Autodesk Fusion 360 part; units mm, degrees
(part 4 of 6)
  spline S19 degree 5 poles (-5.187272, -5.31052) (-5.191544, -5.314884) (-5.200224, -5.323457) (-5.213657, -5.335855) (-5.232349, -5.351511) (-5.256791, -5.369886) (-5.282015, -5.387403) (-5.307733, -5.404393) (-5.333731, -5.421097) (-5.359927, -5.437601) (-5.386324, -5.453892) (-5.412978, -5.469894) (-5.43996, -5.485516) (-5.467316, -5.500697) (-5.495045, -5.515434) (-5.523115, -5.52976) (-5.551479, -5.543728) (-5.580091, -5.55739) (-5.608915, -5.570786) (-5.637941, -5.583924) (-5.66717, -5.5968) (-5.69661, -5.609401) (-5.726271, -5.62171) (-5.756158, -5.633722) (-5.786265, -5.645438) (-5.816583, -5.656867) (-5.847101, -5.66802) (-5.877807, -5.678908) (-5.908693, -5.68954) (-5.939754, -5.699917) (-5.970988, -5.710041) (-6.002394, -5.71991) (-6.033972, -5.729522) (-6.065719, -5.738877) (-6.097633, -5.747977) (-6.129708, -5.756824) (-6.161942, -5.765422) (-6.194329, -5.773774) (-6.226867, -5.781881) (-6.259551, -5.789746) (-6.29238, -5.797368) (-6.325351, -5.804749) (-6.358463, -5.811889) (-6.391713, -5.818788) (-6.425099, -5.825448) (-6.458619, -5.831869) (-6.492269, -5.838053) (-6.526047, -5.844) (-6.55995, -5.849713) (-6.593977, -5.855191) (-6.628126, -5.860435) (-6.662394, -5.865445) (-6.69678, -5.870223) (-6.731281, -5.874768) (-6.765896, -5.879082) (-6.800622, -5.883164) (-6.835457, -5.887016) (-6.8704, -5.890638) (-6.905448, -5.89403) (-6.940601, -5.897193) (-6.975855, -5.900127) (-7.01121, -5.902834) (-7.046664, -5.905312) (-7.082214, -5.907563) (-7.117859, -5.909587) (-7.153598, -5.911384) (-7.189427, -5.912955) (-7.225345, -5.914299) (-7.26135, -5.915418) (-7.297442, -5.916311) (-7.33362, -5.916979) (-7.36263, -5.917334) (-7.384427, -5.917499) (-7.398975, -5.917564) (-7.406253, -5.917586) knots 0 0 0 0 0 0 0.01428571 0.02857143 0.04285714 0.05714286 0.07142857 0.08571429 0.1 0.11428571 0.12857143 0.14285714 0.15714286 0.17142857 0.18571429 0.2 0.21428571 0.22857143 0.24285714 0.25714286 0.27142857 0.28571429 0.3 0.31428571 0.32857143 0.34285714 0.35714286 0.37142857 0.38571429 0.4 0.41428571 0.42857143 0.44285714 0.45714286 0.47142857 0.48571429 0.5 0.51428571 0.52857143 0.54285714 0.55714286 0.57142857 0.58571429 0.6 0.61428571 0.62857143 0.64285714 0.65714286 0.67142857 0.68571429 0.7 0.71428571 0.72857143 0.74285714 0.75714286 0.77142857 0.78571429 0.8 0.81428571 0.82857143 0.84285714 0.85714286 0.87142857 0.88571429 0.9 0.91428571 0.92857143 0.94285714 0.95714286 0.97142857 0.98571429 1 1 1 1 1 1
  line L19 (-5.187272, -5.31052) -> (-4.296111, -4.400225)
  arc A39 (-4.018202, -4.392567) -> (-4.296111, -4.400225) centre (-4.153195, -4.540136) ccw
  arc A40 (-4.018202, -4.392567) -> (-2.935886, -5.178915) centre (0, 0) ccw
  circle A41 centre (0, 0) radius 12.5
  line L20 (0, 0) -> (0, 10)
  circle A42 centre (0, 10) radius 1.1
  circle A43 centre (-9.510565, 3.09017) radius 1.1
  circle A44 centre (-5.877853, -8.09017) radius 1.1
  circle A45 centre (5.877853, -8.09017) radius 1.1
  circle A46 centre (9.510565, 3.09017) radius 1.1
  dimension "d32" = 25
  dimension "d33" = 2.2
  dimension "d35" = 360
  constraint coincident A0.centre A2.centre
  constraint vertical L20
  constraint coincident L20.end A42.centre
  measures "d32" diameter of A41
  measures "d33" diameter of A42
extrude "押し出し4" add sketch "スケッチ3 (2)" along normal blind 3 contours A1 L0 S0 A2 S1 L1 A3 A4 A5 L2 S2 A6 S3 L3 A7 A8 A9 L4 S4 A10 S5 L5 A11 A12 A13 L6 S6 A14 S7 L7 A15 A16 A17 L8 S8 A18 S9 L9 A19 A20 A21 L10 S10 A22 S11 L11 A23 A24 A25 L12 S12 A26 S13 L13 A27 A28 A29 L14 S14 A30 S15 L15 A31 A32 A33 L16 S16 A34 S17 L17 A35 A36 A37 L18 S18 A38 S19 L19 A39 A40 | A41 picked at (1.494301, -4.858237) picked at (-9.44973, -3.004865) in component "Spur Gear (10 teeth)"
sketch "スケッチ4" plane through (0, 0, 0) normal (0, 0, 1) x (1, 0, 0)
  circle A0 centre (0, 0) radius 12.5
  circle A1 centre (-5.877853, -8.09017) radius 1.1
  circle A2 centre (5.877853, -8.09017) radius 1.1
  circle A3 centre (0, 10) radius 1.1
  circle A4 centre (-9.510565, 3.09017) radius 1.1
  circle A5 centre (9.510565, 3.09017) radius 1.1
  arc A6 (6.062014, -1.034666) -> (5.83268, -1.191821) centre (6.028631, -1.231861) ccw
  arc A7 (5.419272, -2.46416) -> (5.83268, -1.191821) centre (0, 0) ccw
  arc A8 (5.419272, -2.46416) -> (5.512434, -2.7261) centre (5.601334, -2.546944) ccw
  line L0 (5.512434, -2.7261) -> (6.65356, -3.292348)
  spline S0 degree 5 poles (6.65356, -3.292348) (6.65903, -3.295062) (6.669866, -3.300669) (6.685809, -3.309612) (6.706474, -3.322552) (6.731503, -3.340119) (6.755957, -3.358695) (6.780063, -3.377904) (6.803983, -3.397468) (6.827775, -3.417282) (6.851425, -3.437354) (6.87488, -3.457758) (6.898076, -3.478592) (6.920967, -3.499918) (6.943552, -3.521735) (6.965851, -3.544004) (6.9879, -3.566665) (7.009735, -3.589654) (7.031382, -3.612928) (7.052847, -3.636473) (7.074125, -3.660292) (7.095206, -3.684398) (7.116079, -3.708803) (7.136739, -3.733515) (7.157185, -3.758529) (7.177423, -3.783831) (7.197461, -3.809409) (7.217305, -3.835248) (7.23696, -3.861337) (7.256428, -3.887671) (7.275709, -3.914247) (7.294799, -3.941067) (7.313699, -3.968129) (7.332406, -3.995431) (7.350923, -4.022971) (7.369249, -4.050743) (7.387387, -4.078742) (7.405338, -4.106963) (7.423103, -4.135402) (7.440683, -4.164057) (7.458077, -4.192923) (7.475285, -4.222) (7.492308, -4.251285) (7.509144, -4.280776) (7.525795, -4.31047) (7.54226, -4.340365) (7.55854, -4.370457) (7.574634, -4.400744) (7.590544, -4.431223) (7.606268, -4.461892) (7.621808, -4.492749) (7.637163, -4.523791) (7.652332, -4.555018) (7.667317, -4.586426) (7.682116, -4.618013) (7.696729, -4.649778) (7.711157, -4.681718) (7.7254, -4.713832) (7.739456, -4.746116) (7.753327, -4.778571) (7.767012, -4.811193) (7.780512, -4.843981) (7.793825, -4.876933) (7.806951, -4.910048) (7.819891, -4.943324) (7.832644, -4.976757) (7.845209, -5.010347) (7.857587, -5.044092) (7.869777, -5.07799) (7.881779, -5.112039) (7.893594, -5.14624) (7.902897, -5.173721) (7.909789, -5.194399) (7.914347, -5.208215) (7.916616, -5.21513) knots 0 0 0 0 0 0 0.01428571 0.02857143 0.04285714 0.05714286 0.07142857 0.08571429 0.1 0.11428571 0.12857143 0.14285714 0.15714286 0.17142857 0.18571429 0.2 0.21428571 0.22857143 0.24285714 0.25714286 0.27142857 0.28571429 0.3 0.31428571 0.32857143 0.34285714 0.35714286 0.37142857 0.38571429 0.4 0.41428571 0.42857143 0.44285714 0.45714286 0.47142857 0.48571429 0.5 0.51428571 0.52857143 0.54285714 0.55714286 0.57142857 0.58571429 0.6 0.61428571 0.62857143 0.64285714 0.65714286 0.67142857 0.68571429 0.7 0.71428571 0.72857143 0.74285714 0.75714286 0.77142857 0.78571429 0.8 0.81428571 0.82857143 0.84285714 0.85714286 0.87142857 0.88571429 0.9 0.91428571 0.92857143 0.94285714 0.95714286 0.97142857 0.98571429 1 1 1 1 1 1
  arc A9 (7.406253, -5.917586) -> (7.916616, -5.21513) centre (0, 0) ccw
  spline S1 degree 5 poles (5.187272, -5.31052) (5.191544, -5.314884) (5.200224, -5.323457) (5.213657, -5.335855) (5.232349, -5.351511) (5.256791, -5.369886) (5.282015, -5.387403) (5.307733, -5.404393) (5.333731, -5.421097) (5.359927, -5.437601) (5.386324, -5.453892) (5.412978, -5.469894) (5.43996, -5.485516) (5.467316, -5.500697) (5.495045, -5.515434) (5.523115, -5.52976) (5.551479, -5.543728) (5.580091, -5.55739) (5.608915, -5.570786) (5.637941, -5.583924) (5.66717, -5.5968) (5.69661, -5.609401) (5.726271, -5.62171) (5.756158, -5.633722) (5.786265, -5.645438) (5.816583, -5.656867) (5.847101, -5.66802) (5.877807, -5.678908) (5.908693, -5.68954) (5.939754, -5.699917) (5.970988, -5.710041) (6.002394, -5.71991) (6.033972, -5.729522) (6.065719, -5.738877) (6.097633, -5.747977) (6.129708, -5.756824) (6.161942, -5.765422) (6.194329, -5.773774) (6.226867, -5.781881) (6.259551, -5.789746) (6.29238, -5.797368) (6.325351, -5.804749) (6.358463, -5.811889) (6.391713, -5.818788) (6.425099, -5.825448) (6.458619, -5.831869) (6.492269, -5.838053) (6.526047, -5.844) (6.55995, -5.849713) (6.593977, -5.855191) (6.628126, -5.860435) (6.662394, -5.865445) (6.69678, -5.870223) (6.731281, -5.874768) (6.765896, -5.879082) (6.800622, -5.883164) (6.835457, -5.887016) (6.8704, -5.890638) (6.905448, -5.89403) (6.940601, -5.897193) (6.975855, -5.900127) (7.01121, -5.902834) (7.046664, -5.905312) (7.082214, -5.907563) (7.117859, -5.909587) (7.153598, -5.911384) (7.189427, -5.912955) (7.225345, -5.914299) (7.26135, -5.915418) (7.297442, -5.916311) (7.33362, -5.916979) (7.36263, -5.917334) (7.384427, -5.917499) (7.398975, -5.917564) (7.406253, -5.917586) knots 0 0 0 0 0 0 0.01428571 0.02857143 0.04285714 0.05714286 0.07142857 0.08571429 0.1 0.11428571 0.12857143 0.14285714 0.15714286 0.17142857 0.18571429 0.2 0.21428571 0.22857143 0.24285714 0.25714286 0.27142857 0.28571429 0.3 0.31428571 0.32857143 0.34285714 0.35714286 0.37142857 0.38571429 0.4 0.41428571 0.42857143 0.44285714 0.45714286 0.47142857 0.48571429 0.5 0.51428571 0.52857143 0.54285714 0.55714286 0.57142857 0.58571429 0.6 0.61428571 0.62857143 0.64285714 0.65714286 0.67142857 0.68571429 0.7 0.71428571 0.72857143 0.74285714 0.75714286 0.77142857 0.78571429 0.8 0.81428571 0.82857143 0.84285714 0.85714286 0.87142857 0.88571429 0.9 0.91428571 0.92857143 0.94285714 0.95714286 0.97142857 0.98571429 1 1 1 1 1 1
  line L1 (5.187272, -5.31052) -> (4.296111, -4.400225)
  arc A10 (4.296111, -4.400225) -> (4.018202, -4.392567) centre (4.153195, -4.540136) ccw
  arc A11 (2.935886, -5.178915) -> (4.018202, -4.392567) centre (0, 0) ccw
  arc A12 (2.935886, -5.178915) -> (2.857291, -5.445588) centre (3.034518, -5.352903) ccw
  line L2 (2.857291, -5.445588) -> (3.44765, -6.57443)
  spline S2 degree 5 poles (3.44765, -6.57443) (3.450479, -6.579841) (3.45595, -6.590746) (3.463592, -6.607352) (3.472705, -6.629968) (3.482628, -6.658891) (3.491493, -6.688294) (3.499704, -6.718003) (3.507556, -6.747891) (3.515158, -6.777905) (3.522493, -6.808044) (3.529476, -6.838338) (3.535996, -6.868827) (3.54198, -6.899536) (3.547427, -6.930461) (3.552378, -6.961584) (3.556897, -6.992877) (3.56105, -7.02431) (3.564882, -7.055863) (3.568408, -7.087528) (3.571621, -7.119305) (3.574508, -7.151198) (3.577049, -7.183212) (3.579237, -7.215347) (3.581076, -7.247601) (3.582577, -7.279967) (3.583753, -7.312438) (3.58462, -7.345006) (3.585187, -7.377666) (3.585459, -7.410413) (3.585435, -7.443247) (3.585115, -7.476166) (3.584499, -7.509168) (3.583586, -7.542252) (3.582378, -7.575416) (3.580881, -7.608656) (3.579097, -7.641969) (3.577032, -7.675351) (3.574688, -7.708802) (3.572068, -7.742316) (3.569173, -7.775894) (3.566003, -7.809533) (3.562562, -7.84323) (3.558848, -7.876985) (3.554865, -7.910795) (3.550614, -7.944658) (3.546097, -7.978572) (3.541315, -8.012535) (3.536271, -8.046544) (3.530966, -8.080599) (3.525401, -8.114697) (3.519577, -8.148836) (3.513495, -8.183015) (3.507156, -8.217232) (3.500562, -8.251486) (3.493714, -8.285774) (3.486612, -8.320094) (3.479259, -8.354446) (3.471655, -8.388827) (3.4638, -8.423236) (3.455697, -8.457672) (3.447346, -8.492133) (3.438747, -8.526617) (3.429902, -8.561123) (3.420812, -8.59565) (3.411477, -8.630194) (3.401899, -8.664755) (3.392078, -8.69933) (3.382016, -8.733919) (3.371712, -8.76852) (3.361168, -8.803134) (3.352541, -8.830834) (3.345963, -8.851615) (3.341529, -8.865471) (3.3393, -8.872399) knots 0 0 0 0 0 0 0.01428571 0.02857143 0.04285714 0.05714286 0.07142857 0.08571429 0.1 0.11428571 0.12857143 0.14285714 0.15714286 0.17142857 0.18571429 0.2 0.21428571 0.22857143 0.24285714 0.25714286 0.27142857 0.28571429 0.3 0.31428571 0.32857143 0.34285714 0.35714286 0.37142857 0.38571429 0.4 0.41428571 0.42857143 0.44285714 0.45714286 0.47142857 0.48571429 0.5 0.51428571 0.52857143 0.54285714 0.55714286 0.57142857 0.58571429 0.6 0.61428571 0.62857143 0.64285714 0.65714286 0.67142857 0.68571429 0.7 0.71428571 0.72857143 0.74285714 0.75714286 0.77142857 0.78571429 0.8 0.81428571 0.82857143 0.84285714 0.85714286 0.87142857 0.88571429 0.9 0.91428571 0.92857143 0.94285714 0.95714286 0.97142857 0.98571429 1 1 1 1 1 1
  arc A13 (2.513515, -9.140714) -> (3.3393, -8.872399) centre (0, 0) ccw
  spline S3 degree 5 poles (1.075146, -7.345303) (1.076037, -7.351344) (1.078021, -7.363382) (1.0816, -7.381308) (1.08752, -7.404961) (1.096493, -7.434193) (1.106603, -7.463191) (1.117423, -7.492053) (1.128638, -7.520848) (1.14013, -7.549598) (1.151911, -7.578293) (1.164069, -7.606906) (1.176715, -7.635404) (1.189923, -7.663765) (1.203694, -7.691986) (1.217982, -7.720075) (1.23272, -7.748048) (1.247836, -7.775918) (1.263282, -7.803698) (1.279042, -7.831388) (1.29512, -7.858985) (1.311531, -7.886484) (1.328292, -7.913877) (1.345411, -7.941161) (1.362881, -7.968336) (1.380692, -7.995403) (1.398826, -8.022364) (1.417268, -8.049222) (1.436006, -8.075977) (1.455035, -8.10263) (1.474353, -8.129179) (1.493961, -8.155623) (1.513858, -8.18196) (1.534043, -8.208189) (1.554513, -8.234309) (1.575262, -8.260321) (1.596286, -8.286223) (1.617579, -8.312017) (1.639136, -8.3377) (1.660956, -8.363274) (1.683035, -8.388737) (1.705371, -8.414089) (1.727962, -8.439328) (1.750807, -8.464453) (1.773902, -8.489465) (1.797246, -8.514362) (1.820834, -8.539144) (1.844665, -8.56381) (1.868736, -8.588359) (1.893045, -8.612791) (1.91759, -8.637106) (1.942368, -8.661302) (1.967379, -8.685379) (1.992619, -8.709335) (2.018087, -8.733171) (2.043782, -8.756885) (2.0697, -8.780477) (2.095841, -8.803946) (2.122201, -8.827291) (2.148781, -8.850512) (2.175577, -8.873608) (2.202589, -8.896579) (2.229815, -8.919423) (2.257253, -8.94214) (2.284901, -8.964729) (2.312758, -8.98719) (2.340821, -9.00952) (2.369089, -9.031719) (2.39756, -9.053788) (2.426234, -9.075725) (2.45511, -9.09753) (2.478372, -9.114869) (2.495908, -9.127814) (2.507639, -9.136418) (2.513515, -9.140714) knots 0 0 0 0 0 0 0.01428571 0.02857143 0.04285714 0.05714286 0.07142857 0.08571429 0.1 0.11428571 0.12857143 0.14285714 0.15714286 0.17142857 0.18571429 0.2 0.21428571 0.22857143 0.24285714 0.25714286 0.27142857 0.28571429 0.3 0.31428571 0.32857143 0.34285714 0.35714286 0.37142857 0.38571429 0.4 0.41428571 0.42857143 0.44285714 0.45714286 0.47142857 0.48571429 0.5 0.51428571 0.52857143 0.54285714 0.55714286 0.57142857 0.58571429 0.6 0.61428571 0.62857143 0.64285714 0.65714286 0.67142857 0.68571429 0.7 0.71428571 0.72857143 0.74285714 0.75714286 0.77142857 0.78571429 0.8 0.81428571 0.82857143 0.84285714 0.85714286 0.87142857 0.88571429 0.9 0.91428571 0.92857143 0.94285714 0.95714286 0.97142857 0.98571429 1 1 1 1 1 1
  line L3 (1.075146, -7.345303) -> (0.889239, -6.085047)
  arc A14 (0.889239, -6.085047) -> (0.668908, -5.915501) centre (0.69138, -6.114234) ccw
  arc A15 (-0.668908, -5.915501) -> (0.668908, -5.915501) centre (0, 0) ccw
  arc A16 (-0.668908, -5.915501) -> (-0.889239, -6.085047) centre (-0.69138, -6.114234) ccw
  line L4 (-0.889239, -6.085047) -> (-1.075146, -7.345303)
  spline S4 degree 5 poles (-1.075146, -7.345303) (-1.076037, -7.351344) (-1.078021, -7.363382) (-1.0816, -7.381308) (-1.08752, -7.404961) (-1.096493, -7.434193) (-1.106603, -7.463191) (-1.117423, -7.492053) (-1.128638, -7.520848) (-1.14013, -7.549598) (-1.151911, -7.578293) (-1.164069, -7.606906) (-1.176715, -7.635404) (-1.189923, -7.663765) (-1.203694, -7.691986) (-1.217982, -7.720075) (-1.23272, -7.748048) (-1.247836, -7.775918) (-1.263282, -7.803698) (-1.279042, -7.831388) (-1.29512, -7.858985) (-1.311531, -7.886484) (-1.328292, -7.913877) (-1.345411, -7.941161) (-1.362881, -7.968336) (-1.380692, -7.995403) (-1.398826, -8.022364) (-1.417268, -8.049222) (-1.436006, -8.075977) (-1.455035, -8.10263) (-1.474353, -8.129179) (-1.493961, -8.155623) (-1.513858, -8.18196) (-1.534043, -8.208189) (-1.554513, -8.234309) (-1.575262, -8.260321) (-1.596286, -8.286223) (-1.617579, -8.312017) (-1.639136, -8.3377) (-1.660956, -8.363274) (-1.683035, -8.388737) (-1.705371, -8.414089) (-1.727962, -8.439328) (-1.750807, -8.464453) (-1.773902, -8.489465) (-1.797246, -8.514362) (-1.820834, -8.539144) (-1.844665, -8.56381) (-1.868736, -8.588359) (-1.893045, -8.612791) (-1.91759, -8.637106) (-1.942368, -8.661302) (-1.967379, -8.685379) (-1.992619, -8.709335) (-2.018087, -8.733171) (-2.043782, -8.756885) (-2.0697, -8.780477) (-2.095841, -8.803946) (-2.122201, -8.827291) (-2.148781, -8.850512) (-2.175577, -8.873608) (-2.202589, -8.896579) (-2.229815, -8.919423) (-2.257253, -8.94214) (-2.284901, -8.964729) (-2.312758, -8.98719) (-2.340821, -9.00952) (-2.369089, -9.031719) (-2.39756, -9.053788) (-2.426234, -9.075725) (-2.45511, -9.09753) (-2.478372, -9.114869) (-2.495908, -9.127814) (-2.507639, -9.136418) (-2.513515, -9.140714) knots 0 0 0 0 0 0 0.01428571 0.02857143 0.04285714 0.05714286 0.07142857 0.08571429 0.1 0.11428571 0.12857143 0.14285714 0.15714286 0.17142857 0.18571429 0.2 0.21428571 0.22857143 0.24285714 0.25714286 0.27142857 0.28571429 0.3 0.31428571 0.32857143 0.34285714 0.35714286 0.37142857 0.38571429 0.4 0.41428571 0.42857143 0.44285714 0.45714286 0.47142857 0.48571429 0.5 0.51428571 0.52857143 0.54285714 0.55714286 0.57142857 0.58571429 0.6 0.61428571 0.62857143 0.64285714 0.65714286 0.67142857 0.68571429 0.7 0.71428571 0.72857143 0.74285714 0.75714286 0.77142857 0.78571429 0.8 0.81428571 0.82857143 0.84285714 0.85714286 0.87142857 0.88571429 0.9 0.91428571 0.92857143 0.94285714 0.95714286 0.97142857 0.98571429 1 1 1 1 1 1
  arc A17 (-3.3393, -8.872399) -> (-2.513515, -9.140714) centre (0, 0) ccw
  spline S5 degree 5 poles (-3.44765, -6.57443) (-3.450479, -6.579841) (-3.45595, -6.590746) (-3.463592, -6.607352) (-3.472705, -6.629968) (-3.482628, -6.658891) (-3.491493, -6.688294) (-3.499704, -6.718003) (-3.507556, -6.747891) (-3.515158, -6.777905) (-3.522493, -6.808044) (-3.529476, -6.838338) (-3.535996, -6.868827) (-3.54198, -6.899536) (-3.547427, -6.930461) (-3.552378, -6.961584) (-3.556897, -6.992877) (-3.56105, -7.02431) (-3.564882, -7.055863) (-3.568408, -7.087528) (-3.571621, -7.119305) (-3.574508, -7.151198) (-3.577049, -7.183212) (-3.579237, -7.215347) (-3.581076, -7.247601) (-3.582577, -7.279967) (-3.583753, -7.312438) (-3.58462, -7.345006) (-3.585187, -7.377666) (-3.585459, -7.410413) (-3.585435, -7.443247) (-3.585115, -7.476166) (-3.584499, -7.509168) (-3.583586, -7.542252) (-3.582378, -7.575416) (-3.580881, -7.608656) (-3.579097, -7.641969) (-3.577032, -7.675351) (-3.574688, -7.708802) (-3.572068, -7.742316) (-3.569173, -7.775894) (-3.566003, -7.809533) (-3.562562, -7.84323) (-3.558848, -7.876985) (-3.554865, -7.910795) (-3.550614, -7.944658) (-3.546097, -7.978572) (-3.541315, -8.012535) (-3.536271, -8.046544) (-3.530966, -8.080599) (-3.525401, -8.114697) (-3.519577, -8.148836) (-3.513495, -8.183015) (-3.507156, -8.217232) (-3.500562, -8.251486) (-3.493714, -8.285774) (-3.486612, -8.320094) (-3.479259, -8.354446) (-3.471655, -8.388827) (-3.4638, -8.423236) (-3.455697, -8.457672) (-3.447346, -8.492133) (-3.438747, -8.526617) (-3.429902, -8.561123) (-3.420812, -8.59565) (-3.411477, -8.630194) (-3.401899, -8.664755) (-3.392078, -8.69933) (-3.382016, -8.733919) (-3.371712, -8.76852) (-3.361168, -8.803134) (-3.352541, -8.830834) (-3.345963, -8.851615) (-3.341529, -8.865471) (-3.3393, -8.872399) knots 0 0 0 0 0 0 0.01428571 0.02857143 0.04285714 0.05714286 0.07142857 0.08571429 0.1 0.11428571 0.12857143 0.14285714 0.15714286 0.17142857 0.18571429 0.2 0.21428571 0.22857143 0.24285714 0.25714286 0.27142857 0.28571429 0.3 0.31428571 0.32857143 0.34285714 0.35714286 0.37142857 0.38571429 0.4 0.41428571 0.42857143 0.44285714 0.45714286 0.47142857 0.48571429 0.5 0.51428571 0.52857143 0.54285714 0.55714286 0.57142857 0.58571429 0.6 0.61428571 0.62857143 0.64285714 0.65714286 0.67142857 0.68571429 0.7 0.71428571 0.72857143 0.74285714 0.75714286 0.77142857 0.78571429 0.8 0.81428571 0.82857143 0.84285714 0.85714286 0.87142857 0.88571429 0.9 0.91428571 0.92857143 0.94285714 0.95714286 0.97142857 0.98571429 1 1 1 1 1 1
  line L5 (-3.44765, -6.57443) -> (-2.857291, -5.445588)
  arc A18 (-2.857291, -5.445588) -> (-2.935886, -5.178915) centre (-3.034518, -5.352903) ccw
  arc A19 (-4.018202, -4.392567) -> (-2.935886, -5.178915) centre (0, 0) ccw
  arc A20 (-4.018202, -4.392567) -> (-4.296111, -4.400225) centre (-4.153195, -4.540136) ccw
  line L6 (-4.296111, -4.400225) -> (-5.187272, -5.31052)
  spline S6 degree 5 poles (-5.187272, -5.31052) (-5.191544, -5.314884) (-5.200224, -5.323457) (-5.213657, -5.335855) (-5.232349, -5.351511) (-5.256791, -5.369886) (-5.282015, -5.387403) (-5.307733, -5.404393) (-5.333731, -5.421097) (-5.359927, -5.437601) (-5.386324, -5.453892) (-5.412978, -5.469894) (-5.43996, -5.485516) (-5.467316, -5.500697) (-5.495045, -5.515434) (-5.523115, -5.52976) (-5.551479, -5.543728) (-5.580091, -5.55739) (-5.608915, -5.570786) (-5.637941, -5.583924) (-5.66717, -5.5968) (-5.69661, -5.609401) (-5.726271, -5.62171) (-5.756158, -5.633722) (-5.786265, -5.645438) (-5.816583, -5.656867) (-5.847101, -5.66802) (-5.877807, -5.678908) (-5.908693, -5.68954) (-5.939754, -5.699917) (-5.970988, -5.710041) (-6.002394, -5.71991) (-6.033972, -5.729522) (-6.065719, -5.738877) (-6.097633, -5.747977) (-6.129708, -5.756824) (-6.161942, -5.765422) (-6.194329, -5.773774) (-6.226867, -5.781881) (-6.259551, -5.789746) (-6.29238, -5.797368) (-6.325351, -5.804749) (-6.358463, -5.811889) (-6.391713, -5.818788) (-6.425099, -5.825448) (-6.458619, -5.831869) (-6.492269, -5.838053) (-6.526047, -5.844) (-6.55995, -5.849713) (-6.593977, -5.855191) (-6.628126, -5.860435) (-6.662394, -5.865445) (-6.69678, -5.870223) (-6.731281, -5.874768) (-6.765896, -5.879082) (-6.800622, -5.883164) (-6.835457, -5.887016) (-6.8704, -5.890638) (-6.905448, -5.89403) (-6.940601, -5.897193) (-6.975855, -5.900127) (-7.01121, -5.902834) (-7.046664, -5.905312) (-7.082214, -5.907563) (-7.117859, -5.909587) (-7.153598, -5.911384) (-7.189427, -5.912955) (-7.225345, -5.914299) (-7.26135, -5.915418) (-7.297442, -5.916311) (-7.33362, -5.916979) (-7.36263, -5.917334) (-7.384427, -5.917499) (-7.398975, -5.917564) (-7.406253, -5.917586) knots 0 0 0 0 0 0 0.01428571 0.02857143 0.04285714 0.05714286 0.07142857 0.08571429 0.1 0.11428571 0.12857143 0.14285714 0.15714286 0.17142857 0.18571429 0.2 0.21428571 0.22857143 0.24285714 0.25714286 0.27142857 0.28571429 0.3 0.31428571 0.32857143 0.34285714 0.35714286 0.37142857 0.38571429 0.4 0.41428571 0.42857143 0.44285714 0.45714286 0.47142857 0.48571429 0.5 0.51428571 0.52857143 0.54285714 0.55714286 0.57142857 0.58571429 0.6 0.61428571 0.62857143 0.64285714 0.65714286 0.67142857 0.68571429 0.7 0.71428571 0.72857143 0.74285714 0.75714286 0.77142857 0.78571429 0.8 0.81428571 0.82857143 0.84285714 0.85714286 0.87142857 0.88571429 0.9 0.91428571 0.92857143 0.94285714 0.95714286 0.97142857 0.98571429 1 1 1 1 1 1
  arc A21 (-7.916616, -5.21513) -> (-7.406253, -5.917586) centre (0, 0) ccw
  spline S7 degree 5 poles (-6.65356, -3.292348) (-6.65903, -3.295062) (-6.669866, -3.300669) (-6.685809, -3.309612) (-6.706474, -3.322552) (-6.731503, -3.340119) (-6.755957, -3.358695) (-6.780063, -3.377904) (-6.803983, -3.397468) (-6.827775, -3.417282) (-6.851425, -3.437354) (-6.87488, -3.457758) (-6.898076, -3.478592) (-6.920967, -3.499918) (-6.943552, -3.521735) (-6.965851, -3.544004) (-6.9879, -3.566665) (-7.009735, -3.589654) (-7.031382, -3.612928) (-7.052847, -3.636473) (-7.074125, -3.660292) (-7.095206, -3.684398) (-7.116079, -3.708803) (-7.136739, -3.733515) (-7.157185, -3.758529) (-7.177423, -3.783831) (-7.197461, -3.809409) (-7.217305, -3.835248) (-7.23696, -3.861337) (-7.256428, -3.887671) (-7.275709, -3.914247) (-7.294799, -3.941067) (-7.313699, -3.968129) (-7.332406, -3.995431) (-7.350923, -4.022971) (-7.369249, -4.050743) (-7.387387, -4.078742) (-7.405338, -4.106963) (-7.423103, -4.135402) (-7.440683, -4.164057) (-7.458077, -4.192923) (-7.475285, -4.222) (-7.492308, -4.251285) (-7.509144, -4.280776) (-7.525795, -4.31047) (-7.54226, -4.340365) (-7.55854, -4.370457) (-7.574634, -4.400744) (-7.590544, -4.431223) (-7.606268, -4.461892) (-7.621808, -4.492749) (-7.637163, -4.523791) (-7.652332, -4.555018) (-7.667317, -4.586426) (-7.682116, -4.618013) (-7.696729, -4.649778) (-7.711157, -4.681718) (-7.7254, -4.713832) (-7.739456, -4.746116) (-7.753327, -4.778571) (-7.767012, -4.811193) (-7.780512, -4.843981) (-7.793825, -4.876933) (-7.806951, -4.910048) (-7.819891, -4.943324) (-7.832644, -4.976757) (-7.845209, -5.010347) (-7.857587, -5.044092) (-7.869777, -5.07799) (-7.881779, -5.112039) (-7.893594, -5.14624) (-7.902897, -5.173721) (-7.909789, -5.194399) (-7.914347, -5.208215) (-7.916616, -5.21513) knots 0 0 0 0 0 0 0.01428571 0.02857143 0.04285714 0.05714286 0.07142857 0.08571429 0.1 0.11428571 0.12857143 0.14285714 0.15714286 0.17142857 0.18571429 0.2 0.21428571 0.22857143 0.24285714 0.25714286 0.27142857 0.28571429 0.3 0.31428571 0.32857143 0.34285714 0.35714286 0.37142857 0.38571429 0.4 0.41428571 0.42857143 0.44285714 0.45714286 0.47142857 0.48571429 0.5 0.51428571 0.52857143 0.54285714 0.55714286 0.57142857 0.58571429 0.6 0.61428571 0.62857143 0.64285714 0.65714286 0.67142857 0.68571429 0.7 0.71428571 0.72857143 0.74285714 0.75714286 0.77142857 0.78571429 0.8 0.81428571 0.82857143 0.84285714 0.85714286 0.87142857 0.88571429 0.9 0.91428571 0.92857143 0.94285714 0.95714286 0.97142857 0.98571429 1 1 1 1 1 1
  line L7 (-6.65356, -3.292348) -> (-5.512434, -2.7261)
  arc A22 (-5.512434, -2.7261) -> (-5.419272, -2.46416) centre (-5.601334, -2.546944) ccw
  arc A23 (-5.83268, -1.191821) -> (-5.419272, -2.46416) centre (0, 0) ccw
  arc A24 (-5.83268, -1.191821) -> (-6.062014, -1.034666) centre (-6.028631, -1.231861) ccw
  line L8 (-6.062014, -1.034666) -> (-7.318037, -1.247299)
  spline S8 degree 5 poles (-7.318037, -1.247299) (-7.324057, -1.248318) (-7.336119, -1.250152) (-7.354274, -1.252287) (-7.378599, -1.253966) (-7.409173, -1.254465) (-7.439876, -1.253811) (-7.470669, -1.252439) (-7.50152, -1.250671) (-7.532414, -1.248626) (-7.563345, -1.246289) (-7.594314, -1.243568) (-7.625326, -1.240347) (-7.65638, -1.236549) (-7.687475, -1.232173) (-7.718605, -1.227264) (-7.749763, -1.221892) (-7.78094, -1.216128) (-7.812133, -1.210023) (-7.843338, -1.203591) (-7.874553, -1.196828) (-7.905777, -1.189717) (-7.937009, -1.182242) (-7.968248, -1.174392) (-7.999492, -1.166174) (-8.030737, -1.157599) (-8.061983, -1.148684) (-8.093224, -1.139445) (-8.124461, -1.129892) (-8.155689, -1.12003) (-8.186909, -1.109861) (-8.218118, -1.099385) (-8.249314, -1.088601) (-8.280497, -1.077508) (-8.311664, -1.066112) (-8.342815, -1.054416) (-8.373946, -1.042426) (-8.405057, -1.030146) (-8.436145, -1.01758) (-8.46721, -1.004731) (-8.49825, -0.991601) (-8.529263, -0.978193) (-8.560247, -0.964506) (-8.591203, -0.950544) (-8.622127, -0.936308) (-8.653019, -0.9218) (-8.683877, -0.907024) (-8.7147, -0.891982) (-8.745486, -0.876675) (-8.776235, -0.861106) (-8.806944, -0.845276) (-8.837612, -0.829188) (-8.868239, -0.812841) (-8.898823, -0.796239) (-8.929362, -0.779383) (-8.959856, -0.762274) (-8.990302, -0.744915) (-9.0207, -0.727306) (-9.051049, -0.70945) (-9.081347, -0.691347) (-9.111593, -0.672999) (-9.141787, -0.654407) (-9.171926, -0.635573) (-9.20201, -0.616498) (-9.232037, -0.597184) (-9.262007, -0.577631) (-9.291916, -0.557842) (-9.321764, -0.537818) (-9.351551, -0.517559) (-9.381275, -0.497067) (-9.410936, -0.476343) (-9.434615, -0.459578) (-9.452345, -0.4469) (-9.464153, -0.438402) (-9.470054, -0.434141) knots 0 0 0 0 0 0 0.01428571 0.02857143 0.04285714 0.05714286 0.07142857 0.08571429 0.1 0.11428571 0.12857143 0.14285714 0.15714286 0.17142857 0.18571429 0.2 0.21428571 0.22857143 0.24285714 0.25714286 0.27142857 0.28571429 0.3 0.31428571 0.32857143 0.34285714 0.35714286 0.37142857 0.38571429 0.4 0.41428571 0.42857143 0.44285714 0.45714286 0.47142857 0.48571429 0.5 0.51428571 0.52857143 0.54285714 0.55714286 0.57142857 0.58571429 0.6 0.61428571 0.62857143 0.64285714 0.65714286 0.67142857 0.68571429 0.7 0.71428571 0.72857143 0.74285714 0.75714286 0.77142857 0.78571429 0.8 0.81428571 0.82857143 0.84285714 0.85714286 0.87142857 0.88571429 0.9 0.91428571 0.92857143 0.94285714 0.95714286 0.97142857 0.98571429 1 1 1 1 1 1
  arc A25 (-9.470054, 0.434141) -> (-9.470054, -0.434141) centre (0, 0) ccw
  spline S9 degree 5 poles (-7.318037, 1.247299) (-7.324057, 1.248318) (-7.336119, 1.250152) (-7.354274, 1.252287) (-7.378599, 1.253966) (-7.409173, 1.254465) (-7.439876, 1.253811) (-7.470669, 1.252439) (-7.50152, 1.250671) (-7.532414, 1.248626) (-7.563345, 1.246289) (-7.594314, 1.243568) (-7.625326, 1.240347) (-7.65638, 1.236549) (-7.687475, 1.232173) (-7.718605, 1.227264) (-7.749763, 1.221892) (-7.78094, 1.216128) (-7.812133, 1.210023) (-7.843338, 1.203591) (-7.874553, 1.196828) (-7.905777, 1.189717) (-7.937009, 1.182242) (-7.968248, 1.174392) (-7.999492, 1.166174) (-8.030737, 1.157599) (-8.061983, 1.148684) (-8.093224, 1.139445) (-8.124461, 1.129892) (-8.155689, 1.12003) (-8.186909, 1.109861) (-8.218118, 1.099385) (-8.249314, 1.088601) (-8.280497, 1.077508) (-8.311664, 1.066112) (-8.342815, 1.054416) (-8.373946, 1.042426) (-8.405057, 1.030146) (-8.436145, 1.01758) (-8.46721, 1.004731) (-8.49825, 0.991601) (-8.529263, 0.978193) (-8.560247, 0.964506) (-8.591203, 0.950544) (-8.622127, 0.936308) (-8.653019, 0.9218) (-8.683877, 0.907024) (-8.7147, 0.891982) (-8.745486, 0.876675) (-8.776235, 0.861106) (-8.806944, 0.845276) (-8.837612, 0.829188) (-8.868239, 0.812841) (-8.898823, 0.796239) (-8.929362, 0.779383) (-8.959856, 0.762274) (-8.990302, 0.744915) (-9.0207, 0.727306) (-9.051049, 0.70945) (-9.081347, 0.691347) (-9.111593, 0.672999) (-9.141787, 0.654407) (-9.171926, 0.635573) (-9.20201, 0.616498) (-9.232037, 0.597184) (-9.262007, 0.577631) (-9.291916, 0.557842) (-9.321764, 0.537818) (-9.351551, 0.517559) (-9.381275, 0.497067) (-9.410936, 0.476343) (-9.434615, 0.459578) (-9.452345, 0.4469) (-9.464153, 0.438402) (-9.470054, 0.434141) knots 0 0 0 0 0 0 0.01428571 0.02857143 0.04285714 0.05714286 0.07142857 0.08571429 0.1 0.11428571 0.12857143 0.14285714 0.15714286 0.17142857 0.18571429 0.2 0.21428571 0.22857143 0.24285714 0.25714286 0.27142857 0.28571429 0.3 0.31428571 0.32857143 0.34285714 0.35714286 0.37142857 0.38571429 0.4 0.41428571 0.42857143 0.44285714 0.45714286 0.47142857 0.48571429 0.5 0.51428571 0.52857143 0.54285714 0.55714286 0.57142857 0.58571429 0.6 0.61428571 0.62857143 0.64285714 0.65714286 0.67142857 0.68571429 0.7 0.71428571 0.72857143 0.74285714 0.75714286 0.77142857 0.78571429 0.8 0.81428571 0.82857143 0.84285714 0.85714286 0.87142857 0.88571429 0.9 0.91428571 0.92857143 0.94285714 0.95714286 0.97142857 0.98571429 1 1 1 1 1 1
  line L9 (-7.318037, 1.247299) -> (-6.062014, 1.034666)
  arc A26 (-6.062014, 1.034666) -> (-5.83268, 1.191821) centre (-6.028631, 1.231861) ccw
  arc A27 (-5.419272, 2.46416) -> (-5.83268, 1.191821) centre (0, 0) ccw
  arc A28 (-5.419272, 2.46416) -> (-5.512434, 2.7261) centre (-5.601334, 2.546944) ccw
  line L10 (-5.512434, 2.7261) -> (-6.65356, 3.292348)
  spline S10 degree 5 poles (-6.65356, 3.292348) (-6.65903, 3.295062) (-6.669866, 3.300669) (-6.685809, 3.309612) (-6.706474, 3.322552) (-6.731503, 3.340119) (-6.755957, 3.358695) (-6.780063, 3.377904) (-6.803983, 3.397468) (-6.827775, 3.417282) (-6.851425, 3.437354) (-6.87488, 3.457758) (-6.898076, 3.478592) (-6.920967, 3.499918) (-6.943552, 3.521735) (-6.965851, 3.544004) (-6.9879, 3.566665) (-7.009735, 3.589654) (-7.031382, 3.612928) (-7.052847, 3.636473) (-7.074125, 3.660292) (-7.095206, 3.684398) (-7.116079, 3.708803) (-7.136739, 3.733515) (-7.157185, 3.758529) (-7.177423, 3.783831) (-7.197461, 3.809409) (-7.217305, 3.835248) (-7.23696, 3.861337) (-7.256428, 3.887671) (-7.275709, 3.914247) (-7.294799, 3.941067) (-7.313699, 3.968129) (-7.332406, 3.995431) (-7.350923, 4.022971) (-7.369249, 4.050743) (-7.387387, 4.078742) (-7.405338, 4.106963) (-7.423103, 4.135402) (-7.440683, 4.164057) (-7.458077, 4.192923) (-7.475285, 4.222) (-7.492308, 4.251285) (-7.509144, 4.280776) (-7.525795, 4.31047) (-7.54226, 4.340365) (-7.55854, 4.370457) (-7.574634, 4.400744) (-7.590544, 4.431223) (-7.606268, 4.461892) (-7.621808, 4.492749) (-7.637163, 4.523791) (-7.652332, 4.555018) (-7.667317, 4.586426) (-7.682116, 4.618013) (-7.696729, 4.649778) (-7.711157, 4.681718) (-7.7254, 4.713832) (-7.739456, 4.746116) (-7.753327, 4.778571) (-7.767012, 4.811193) (-7.780512, 4.843981) (-7.793825, 4.876933) (-7.806951, 4.910048) (-7.819891, 4.943324) (-7.832644, 4.976757) (-7.845209, 5.010347) (-7.857587, 5.044092) (-7.869777, 5.07799) (-7.881779, 5.112039) (-7.893594, 5.14624) (-7.902897, 5.173721) (-7.909789, 5.194399) (-7.914347, 5.208215) (-7.916616, 5.21513) knots 0 0 0 0 0 0 0.01428571 0.02857143 0.04285714 0.05714286 0.07142857 0.08571429 0.1 0.11428571 0.12857143 0.14285714 0.15714286 0.17142857 0.18571429 0.2 0.21428571 0.22857143 0.24285714 0.25714286 0.27142857 0.28571429 0.3 0.31428571 0.32857143 0.34285714 0.35714286 0.37142857 0.38571429 0.4 0.41428571 0.42857143 0.44285714 0.45714286 0.47142857 0.48571429 0.5 0.51428571 0.52857143 0.54285714 0.55714286 0.57142857 0.58571429 0.6 0.61428571 0.62857143 0.64285714 0.65714286 0.67142857 0.68571429 0.7 0.71428571 0.72857143 0.74285714 0.75714286 0.77142857 0.78571429 0.8 0.81428571 0.82857143 0.84285714 0.85714286 0.87142857 0.88571429 0.9 0.91428571 0.92857143 0.94285714 0.95714286 0.97142857 0.98571429 1 1 1 1 1 1
  arc A29 (-7.406253, 5.917586) -> (-7.916616, 5.21513) centre (0, 0) ccw
  spline S11 degree 5 poles (-5.187272, 5.31052) (-5.191544, 5.314884) (-5.200224, 5.323457) (-5.213657, 5.335855) (-5.232349, 5.351511) (-5.256791, 5.369886) (-5.282015, 5.387403) (-5.307733, 5.404393) (-5.333731, 5.421097) (-5.359927, 5.437601) (-5.386324, 5.453892) (-5.412978, 5.469894) (-5.43996, 5.485516) (-5.467316, 5.500697) (-5.495045, 5.515434) (-5.523115, 5.52976) (-5.551479, 5.543728) (-5.580091, 5.55739) (-5.608915, 5.570786) (-5.637941, 5.583924) (-5.66717, 5.5968) (-5.69661, 5.609401) (-5.726271, 5.62171) (-5.756158, 5.633722) (-5.786265, 5.645438) (-5.816583, 5.656867) (-5.847101, 5.66802) (-5.877807, 5.678908) (-5.908693, 5.68954) (-5.939754, 5.699917) (-5.970988, 5.710041) (-6.002394, 5.71991) (-6.033972, 5.729522) (-6.065719, 5.738877) (-6.097633, 5.747977) (-6.129708, 5.756824) (-6.161942, 5.765422) (-6.194329, 5.773774) (-6.226867, 5.781881) (-6.259551, 5.789746) (-6.29238, 5.797368) (-6.325351, 5.804749) (-6.358463, 5.811889) (-6.391713, 5.818788) (-6.425099, 5.825448) (-6.458619, 5.831869) (-6.492269, 5.838053) (-6.526047, 5.844) (-6.55995, 5.849713) (-6.593977, 5.855191) (-6.628126, 5.860435) (-6.662394, 5.865445) (-6.69678, 5.870223) (-6.731281, 5.874768) (-6.765896, 5.879082) (-6.800622, 5.883164) (-6.835457, 5.887016) (-6.8704, 5.890638) (-6.905448, 5.89403) (-6.940601, 5.897193) (-6.975855, 5.900127) (-7.01121, 5.902834) (-7.046664, 5.905312) (-7.082214, 5.907563) (-7.117859, 5.909587) (-7.153598, 5.911384) (-7.189427, 5.912955) (-7.225345, 5.914299) (-7.26135, 5.915418) (-7.297442, 5.916311) (-7.33362, 5.916979) (-7.36263, 5.917334) (-7.384427, 5.917499) (-7.398975, 5.917564) (-7.406253, 5.917586) knots 0 0 0 0 0 0 0.01428571 0.02857143 0.04285714 0.05714286 0.07142857 0.08571429 0.1 0.11428571 0.12857143 0.14285714 0.15714286 0.17142857 0.18571429 0.2 0.21428571 0.22857143 0.24285714 0.25714286 0.27142857 0.28571429 0.3 0.31428571 0.32857143 0.34285714 0.35714286 0.37142857 0.38571429 0.4 0.41428571 0.42857143 0.44285714 0.45714286 0.47142857 0.48571429 0.5 0.51428571 0.52857143 0.54285714 0.55714286 0.57142857 0.58571429 0.6 0.61428571 0.62857143 0.64285714 0.65714286 0.67142857 0.68571429 0.7 0.71428571 0.72857143 0.74285714 0.75714286 0.77142857 0.78571429 0.8 0.81428571 0.82857143 0.84285714 0.85714286 0.87142857 0.88571429 0.9 0.91428571 0.92857143 0.94285714 0.95714286 0.97142857 0.98571429 1 1 1 1 1 1
  line L11 (-5.187272, 5.31052) -> (-4.296111, 4.400225)
  arc A30 (-4.296111, 4.400225) -> (-4.018202, 4.392567) centre (-4.153195, 4.540136) ccw
  arc A31 (-2.935886, 5.178915) -> (-4.018202, 4.392567) centre (0, 0) ccw
  arc A32 (-2.935886, 5.178915) -> (-2.857291, 5.445588) centre (-3.034518, 5.352903) ccw
  line L12 (-2.857291, 5.445588) -> (-3.44765, 6.57443)
  spline S12 degree 5 poles (-3.44765, 6.57443) (-3.450479, 6.579841) (-3.45595, 6.590746) (-3.463592, 6.607352) (-3.472705, 6.629968) (-3.482628, 6.658891) (-3.491493, 6.688294) (-3.499704, 6.718003) (-3.507556, 6.747891) (-3.515158, 6.777905) (-3.522493, 6.808044) (-3.529476, 6.838338) (-3.535996, 6.868827) (-3.54198, 6.899536) (-3.547427, 6.930461) (-3.552378, 6.961584) (-3.556897, 6.992877) (-3.56105, 7.02431) (-3.564882, 7.055863) (-3.568408, 7.087528) (-3.571621, 7.119305) (-3.574508, 7.151198) (-3.577049, 7.183212) (-3.579237, 7.215347) (-3.581076, 7.247601) (-3.582577, 7.279967) (-3.583753, 7.312438) (-3.58462, 7.345006) (-3.585187, 7.377666) (-3.585459, 7.410413) (-3.585435, 7.443247) (-3.585115, 7.476166) (-3.584499, 7.509168) (-3.583586, 7.542252) (-3.582378, 7.575416) (-3.580881, 7.608656) (-3.579097, 7.641969) (-3.577032, 7.675351) (-3.574688, 7.708802) (-3.572068, 7.742316) (-3.569173, 7.775894) (-3.566003, 7.809533) (-3.562562, 7.84323) (-3.558848, 7.876985) (-3.554865, 7.910795) (-3.550614, 7.944658) (-3.546097, 7.978572) (-3.541315, 8.012535) (-3.536271, 8.046544) (-3.530966, 8.080599) (-3.525401, 8.114697) (-3.519577, 8.148836) (-3.513495, 8.183015) (-3.507156, 8.217232) (-3.500562, 8.251486) (-3.493714, 8.285774) (-3.486612, 8.320094) (-3.479259, 8.354446) (-3.471655, 8.388827) (-3.4638, 8.423236) (-3.455697, 8.457672) (-3.447346, 8.492133) (-3.438747, 8.526617) (-3.429902, 8.561123) (-3.420812, 8.59565) (-3.411477, 8.630194) (-3.401899, 8.664755) (-3.392078, 8.69933) (-3.382016, 8.733919) (-3.371712, 8.76852) (-3.361168, 8.803134) (-3.352541, 8.830834) (-3.345963, 8.851615) (-3.341529, 8.865471) (-3.3393, 8.872399) knots 0 0 0 0 0 0 0.01428571 0.02857143 0.04285714 0.05714286 0.07142857 0.08571429 0.1 0.11428571 0.12857143 0.14285714 0.15714286 0.17142857 0.18571429 0.2 0.21428571 0.22857143 0.24285714 0.25714286 0.27142857 0.28571429 0.3 0.31428571 0.32857143 0.34285714 0.35714286 0.37142857 0.38571429 0.4 0.41428571 0.42857143 0.44285714 0.45714286 0.47142857 0.48571429 0.5 0.51428571 0.52857143 0.54285714 0.55714286 0.57142857 0.58571429 0.6 0.61428571 0.62857143 0.64285714 0.65714286 0.67142857 0.68571429 0.7 0.71428571 0.72857143 0.74285714 0.75714286 0.77142857 0.78571429 0.8 0.81428571 0.82857143 0.84285714 0.85714286 0.87142857 0.88571429 0.9 0.91428571 0.92857143 0.94285714 0.95714286 0.97142857 0.98571429 1 1 1 1 1 1
  arc A33 (-2.513515, 9.140714) -> (-3.3393, 8.872399) centre (0, 0) ccw
  spline S13 degree 5 poles (-1.075146, 7.345303) (-1.076037, 7.351344) (-1.078021, 7.363382) (-1.0816, 7.381308) (-1.08752, 7.404961) (-1.096493, 7.434193) (-1.106603, 7.463191) (-1.117423, 7.492053) (-1.128638, 7.520848) (-1.14013, 7.549598) (-1.151911, 7.578293) (-1.164069, 7.606906) (-1.176715, 7.635404) (-1.189923, 7.663765) (-1.203694, 7.691986) (-1.217982, 7.720075) (-1.23272, 7.748048) (-1.247836, 7.775918) (-1.263282, 7.803698) (-1.279042, 7.831388) (-1.29512, 7.858985) (-1.311531, 7.886484) (-1.328292, 7.913877) (-1.345411, 7.941161) (-1.362881, 7.968336) (-1.380692, 7.995403) (-1.398826, 8.022364) (-1.417268, 8.049222) (-1.436006, 8.075977) (-1.455035, 8.10263) (-1.474353, 8.129179) (-1.493961, 8.155623) (-1.513858, 8.18196) (-1.534043, 8.208189) (-1.554513, 8.234309) (-1.575262, 8.260321) (-1.596286, 8.286223) (-1.617579, 8.312017) (-1.639136, 8.3377) (-1.660956, 8.363274) (-1.683035, 8.388737) (-1.705371, 8.414089) (-1.727962, 8.439328) (-1.750807, 8.464453) (-1.773902, 8.489465) (-1.797246, 8.514362) (-1.820834, 8.539144) (-1.844665, 8.56381) (-1.868736, 8.588359) (-1.893045, 8.612791) (-1.91759, 8.637106) (-1.942368, 8.661302) (-1.967379, 8.685379) (-1.992619, 8.709335) (-2.018087, 8.733171) (-2.043782, 8.756885) (-2.0697, 8.780477) (-2.095841, 8.803946) (-2.122201, 8.827291) (-2.148781, 8.850512) (-2.175577, 8.873608) (-2.202589, 8.896579) (-2.229815, 8.919423) (-2.257253, 8.94214) (-2.284901, 8.964729) (-2.312758, 8.98719) (-2.340821, 9.00952) (-2.369089, 9.031719) (-2.39756, 9.053788) (-2.426234, 9.075725) (-2.45511, 9.09753) (-2.478372, 9.114869) (-2.495908, 9.127814) (-2.507639, 9.136418) (-2.513515, 9.140714) knots 0 0 0 0 0 0 0.01428571 0.02857143 0.04285714 0.05714286 0.07142857 0.08571429 0.1 0.11428571 0.12857143 0.14285714 0.15714286 0.17142857 0.18571429 0.2 0.21428571 0.22857143 0.24285714 0.25714286 0.27142857 0.28571429 0.3 0.31428571 0.32857143 0.34285714 0.35714286 0.37142857 0.38571429 0.4 0.41428571 0.42857143 0.44285714 0.45714286 0.47142857 0.48571429 0.5 0.51428571 0.52857143 0.54285714 0.55714286 0.57142857 0.58571429 0.6 0.61428571 0.62857143 0.64285714 0.65714286 0.67142857 0.68571429 0.7 0.71428571 0.72857143 0.74285714 0.75714286 0.77142857 0.78571429 0.8 0.81428571 0.82857143 0.84285714 0.85714286 0.87142857 0.88571429 0.9 0.91428571 0.92857143 0.94285714 0.95714286 0.97142857 0.98571429 1 1 1 1 1 1
  line L13 (-1.075146, 7.345303) -> (-0.889239, 6.085047)
  arc A34 (-0.889239, 6.085047) -> (-0.668908, 5.915501) centre (-0.69138, 6.114234) ccw
  arc A35 (0.668908, 5.915501) -> (-0.668908, 5.915501) centre (0, 0) ccw
  arc A36 (0.668908, 5.915501) -> (0.889239, 6.085047) centre (0.69138, 6.114234) ccw
  line L14 (0.889239, 6.085047) -> (1.075146, 7.345303)
  spline S14 degree 5 poles (1.075146, 7.345303) (1.076037, 7.351344) (1.078021, 7.363382) (1.0816, 7.381308) (1.08752, 7.404961) (1.096493, 7.434193) (1.106603, 7.463191) (1.117423, 7.492053) (1.128638, 7.520848) (1.14013, 7.549598) (1.151911, 7.578293) (1.164069, 7.606906) (1.176715, 7.635404) (1.189923, 7.663765) (1.203694, 7.691986) (1.217982, 7.720075) (1.23272, 7.748048) (1.247836, 7.775918) (1.263282, 7.803698) (1.279042, 7.831388) (1.29512, 7.858985) (1.311531, 7.886484) (1.328292, 7.913877) (1.345411, 7.941161) (1.362881, 7.968336) (1.380692, 7.995403) (1.398826, 8.022364) (1.417268, 8.049222) (1.436006, 8.075977) (1.455035, 8.10263) (1.474353, 8.129179) (1.493961, 8.155623) (1.513858, 8.18196) (1.534043, 8.208189) (1.554513, 8.234309) (1.575262, 8.260321) (1.596286, 8.286223) (1.617579, 8.312017) (1.639136, 8.3377) (1.660956, 8.363274) (1.683035, 8.388737) (1.705371, 8.414089) (1.727962, 8.439328) (1.750807, 8.464453) (1.773902, 8.489465) (1.797246, 8.514362) (1.820834, 8.539144) (1.844665, 8.56381) (1.868736, 8.588359) (1.893045, 8.612791) (1.91759, 8.637106) (1.942368, 8.661302) (1.967379, 8.685379) (1.992619, 8.709335) (2.018087, 8.733171) (2.043782, 8.756885) (2.0697, 8.780477) (2.095841, 8.803946) (2.122201, 8.827291) (2.148781, 8.850512) (2.175577, 8.873608) (2.202589, 8.896579) (2.229815, 8.919423) (2.257253, 8.94214) (2.284901, 8.964729) (2.312758, 8.98719) (2.340821, 9.00952) (2.369089, 9.031719) (2.39756, 9.053788) (2.426234, 9.075725) (2.45511, 9.09753) (2.478372, 9.114869) (2.495908, 9.127814) (2.507639, 9.136418) (2.513515, 9.140714) knots 0 0 0 0 0 0 0.01428571 0.02857143 0.04285714 0.05714286 0.07142857 0.08571429 0.1 0.11428571 0.12857143 0.14285714 0.15714286 0.17142857 0.18571429 0.2 0.21428571 0.22857143 0.24285714 0.25714286 0.27142857 0.28571429 0.3 0.31428571 0.32857143 0.34285714 0.35714286 0.37142857 0.38571429 0.4 0.41428571 0.42857143 0.44285714 0.45714286 0.47142857 0.48571429 0.5 0.51428571 0.52857143 0.54285714 0.55714286 0.57142857 0.58571429 0.6 0.61428571 0.62857143 0.64285714 0.65714286 0.67142857 0.68571429 0.7 0.71428571 0.72857143 0.74285714 0.75714286 0.77142857 0.78571429 0.8 0.81428571 0.82857143 0.84285714 0.85714286 0.87142857 0.88571429 0.9 0.91428571 0.92857143 0.94285714 0.95714286 0.97142857 0.98571429 1 1 1 1 1 1
  arc A37 (3.3393, 8.872399) -> (2.513515, 9.140714) centre (0, 0) ccw
  spline S15 degree 5 poles (3.44765, 6.57443) (3.450479, 6.579841) (3.45595, 6.590746) (3.463592, 6.607352) (3.472705, 6.629968) (3.482628, 6.658891) (3.491493, 6.688294) (3.499704, 6.718003) (3.507556, 6.747891) (3.515158, 6.777905) (3.522493, 6.808044) (3.529476, 6.838338) (3.535996, 6.868827) (3.54198, 6.899536) (3.547427, 6.930461) (3.552378, 6.961584) (3.556897, 6.992877) (3.56105, 7.02431) (3.564882, 7.055863) (3.568408, 7.087528) (3.571621, 7.119305) (3.574508, 7.151198) (3.577049, 7.183212) (3.579237, 7.215347) (3.581076, 7.247601) (3.582577, 7.279967) (3.583753, 7.312438) (3.58462, 7.345006) (3.585187, 7.377666) (3.585459, 7.410413) (3.585435, 7.443247) (3.585115, 7.476166) (3.584499, 7.509168) (3.583586, 7.542252) (3.582378, 7.575416) (3.580881, 7.608656) (3.579097, 7.641969) (3.577032, 7.675351) (3.574688, 7.708802) (3.572068, 7.742316) (3.569173, 7.775894) (3.566003, 7.809533) (3.562562, 7.84323) (3.558848, 7.876985) (3.554865, 7.910795) (3.550614, 7.944658) (3.546097, 7.978572) (3.541315, 8.012535) (3.536271, 8.046544) (3.530966, 8.080599) (3.525401, 8.114697) (3.519577, 8.148836) (3.513495, 8.183015) (3.507156, 8.217232) (3.500562, 8.251486) (3.493714, 8.285774) (3.486612, 8.320094) (3.479259, 8.354446) (3.471655, 8.388827) (3.4638, 8.423236) (3.455697, 8.457672) (3.447346, 8.492133) (3.438747, 8.526617) (3.429902, 8.561123) (3.420812, 8.59565) (3.411477, 8.630194) (3.401899, 8.664755) (3.392078, 8.69933) (3.382016, 8.733919) (3.371712, 8.76852) (3.361168, 8.803134) (3.352541, 8.830834) (3.345963, 8.851615) (3.341529, 8.865471) (3.3393, 8.872399) knots 0 0 0 0 0 0 0.01428571 0.02857143 0.04285714 0.05714286 0.07142857 0.08571429 0.1 0.11428571 0.12857143 0.14285714 0.15714286 0.17142857 0.18571429 0.2 0.21428571 0.22857143 0.24285714 0.25714286 0.27142857 0.28571429 0.3 0.31428571 0.32857143 0.34285714 0.35714286 0.37142857 0.38571429 0.4 0.41428571 0.42857143 0.44285714 0.45714286 0.47142857 0.48571429 0.5 0.51428571 0.52857143 0.54285714 0.55714286 0.57142857 0.58571429 0.6 0.61428571 0.62857143 0.64285714 0.65714286 0.67142857 0.68571429 0.7 0.71428571 0.72857143 0.74285714 0.75714286 0.77142857 0.78571429 0.8 0.81428571 0.82857143 0.84285714 0.85714286 0.87142857 0.88571429 0.9 0.91428571 0.92857143 0.94285714 0.95714286 0.97142857 0.98571429 1 1 1 1 1 1
  line L15 (3.44765, 6.57443) -> (2.857291, 5.445588)
  arc A38 (2.857291, 5.445588) -> (2.935886, 5.178915) centre (3.034518, 5.352903) ccw
  arc A39 (4.018202, 4.392567) -> (2.935886, 5.178915) centre (0, 0) ccw
  arc A40 (4.018202, 4.392567) -> (4.296111, 4.400225) centre (4.153195, 4.540136) ccw
  line L16 (4.296111, 4.400225) -> (5.187272, 5.31052)
  spline S16 degree 5 poles (5.187272, 5.31052) (5.191544, 5.314884) (5.200224, 5.323457) (5.213657, 5.335855) (5.232349, 5.351511) (5.256791, 5.369886) (5.282015, 5.387403) (5.307733, 5.404393) (5.333731, 5.421097) (5.359927, 5.437601) (5.386324, 5.453892) (5.412978, 5.469894) (5.43996, 5.485516) (5.467316, 5.500697) (5.495045, 5.515434) (5.523115, 5.52976) (5.551479, 5.543728) (5.580091, 5.55739) (5.608915, 5.570786) (5.637941, 5.583924) (5.66717, 5.5968) (5.69661, 5.609401) (5.726271, 5.62171) (5.756158, 5.633722) (5.786265, 5.645438) (5.816583, 5.656867) (5.847101, 5.66802) (5.877807, 5.678908) (5.908693, 5.68954) (5.939754, 5.699917) (5.970988, 5.710041) (6.002394, 5.71991) (6.033972, 5.729522) (6.065719, 5.738877) (6.097633, 5.747977) (6.129708, 5.756824) (6.161942, 5.765422) (6.194329, 5.773774) (6.226867, 5.781881) (6.259551, 5.789746) (6.29238, 5.797368) (6.325351, 5.804749) (6.358463, 5.811889) (6.391713, 5.818788) (6.425099, 5.825448) (6.458619, 5.831869) (6.492269, 5.838053) (6.526047, 5.844) (6.55995, 5.849713) (6.593977, 5.855191) (6.628126, 5.860435) (6.662394, 5.865445) (6.69678, 5.870223) (6.731281, 5.874768) (6.765896, 5.879082) (6.800622, 5.883164) (6.835457, 5.887016) (6.8704, 5.890638) (6.905448, 5.89403) (6.940601, 5.897193) (6.975855, 5.900127) (7.01121, 5.902834) (7.046664, 5.905312) (7.082214, 5.907563) (7.117859, 5.909587) (7.153598, 5.911384) (7.189427, 5.912955) (7.225345, 5.914299) (7.26135, 5.915418) (7.297442, 5.916311) (7.33362, 5.916979) (7.36263, 5.917334) (7.384427, 5.917499) (7.398975, 5.917564) (7.406253, 5.917586) knots 0 0 0 0 0 0 0.01428571 0.02857143 0.04285714 0.05714286 0.07142857 0.08571429 0.1 0.11428571 0.12857143 0.14285714 0.15714286 0.17142857 0.18571429 0.2 0.21428571 0.22857143 0.24285714 0.25714286 0.27142857 0.28571429 0.3 0.31428571 0.32857143 0.34285714 0.35714286 0.37142857 0.38571429 0.4 0.41428571 0.42857143 0.44285714 0.45714286 0.47142857 0.48571429 0.5 0.51428571 0.52857143 0.54285714 0.55714286 0.57142857 0.58571429 0.6 0.61428571 0.62857143 0.64285714 0.65714286 0.67142857 0.68571429 0.7 0.71428571 0.72857143 0.74285714 0.75714286 0.77142857 0.78571429 0.8 0.81428571 0.82857143 0.84285714 0.85714286 0.87142857 0.88571429 0.9 0.91428571 0.92857143 0.94285714 0.95714286 0.97142857 0.98571429 1 1 1 1 1 1
  arc A41 (7.916616, 5.21513) -> (7.406253, 5.917586) centre (0, 0) ccw